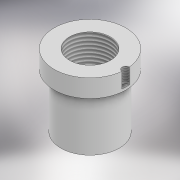
# Autodesk Inventor part: 螺套
Saved by Autodesk Inventor 2020 (Build 240168000, 168)
## iProperties
Created: 2021-04-28
Part Number: 螺套
Material: 常规
Document SubType Name: Modeling
Designer: Luorily
Density: 1 g/cm^3
Appearance: 默认
Author: Luorily
Autodesk Inventor part; units mm, degrees
ref_plane "YZ Plane" through (0, 0, 0) normal (1, 0, 0) x (0, 1, 0)
ref_plane "XZ Plane" through (0, 0, 0) normal (0, 1, 0) x (-1, 0, 0)
ref_plane "XY Plane" through (0, 0, 0) normal (0, 0, 1) x (1, 0, 0)
sketch "草图1" plane through (0, 0, 0) normal (0, 0, 1) x (1, 0, 0)
  line L0 (0, 0) -> (32.5, 0)
  line L1 (32.5, 0) -> (32.5, 60)
  line L2 (32.5, 60) -> (40, 60)
  line L3 (40, 60) -> (40, 80)
  line L4 (40, 80) -> (0, 80)
  line L5 (0, 80) -> (0, 0)
  dimension "d0" = 32.5
  dimension "d1" = 60
  dimension "d2" = 7.5
  dimension "d3" = 20
  constraints: 12 end point, 5 perpendicular, 1 horizontal
  measures "d0" distance of L0.start L0.end
  measures "d1" distance of L0.end L1.end
  measures "d2" distance of L1.end L2.end
  measures "d3" distance of L2.end L3.end
revolve "旋转1" add sketch "草图1" angle 360 about axis through (0, 80, 0) along (0, -1, 0)
sketch "草图2" plane through (0, 80, 0) normal (0, 1, 0) x (1, 0, 0)
  circle A0 centre (0, 0) radius 40 projected
  constraints: 1 coincident
hole "孔1" at (0, 80, 0) direction (0, -1, 0) diameter 45.6699 end through all thread size "M50x4" class "6H" standard "GB Metric profile"
chamfer "倒角1" distance 2 angle 45 1 edges at (0, 0, -22.8349)
sketch "草图3" plane through (0, 80, 0) normal (0, 1, 0) x (1, 0, 0)
  circle A0 centre (0, 0) radius 40 projected
  point P0 (40, 0)
  constraints: 1 horizontal alignment, 1 other
hole "孔2" at (40, 80, 0) direction (0, -1, 0) diameter 8.376 depth 17 thread size "M10x1.5" designation "M10" class "6H" standard "GB Metric profile"
